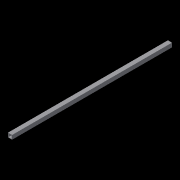
# Autodesk Inventor part: Bumper Rail Side
Saved by Autodesk Inventor 2014 SP1 (Build 180222100, 222)
## iProperties
Created: 2013-11-29
Part Number: Bumper Rail Side
Material: Generic
Document SubType Name: Modeling
Designer: Rauhul Varma
Mass: 82.3834 g
Surface Area: 1040.12 cm^2
Volume: 82.3834 cm^3
Density: 1 g/cm^3
Appearance: Default
Author: Rauhul Varma
Autodesk Inventor part; units mm, degrees
ref_plane "YZ Plane" through (0, 0, 0) normal (1, 0, 0) x (0, 1, 0)
ref_plane "XZ Plane" through (0, 0, 0) normal (0, 1, 0) x (-1, 0, 0)
ref_plane "XY Plane" through (0, 0, 0) normal (0, 0, 1) x (1, 0, 0)
sketch "Sketch1" plane through (0, 0, 0) normal (0, 0, 1) x (1, 0, 0)
  line L0 (0, 0) -> (19.05, 0)
  line L1 (19.05, 0) -> (19.05, 19.05)
  line L2 (19.05, 19.05) -> (0, 19.05)
  line L3 (0, 19.05) -> (0, 0)
  line L4 (17.4625, 17.4625) -> (1.5875, 17.4625)
  line L5 (1.5875, 17.4625) -> (1.5875, 1.5875)
  line L6 (1.5875, 1.5875) -> (17.4625, 1.5875)
  line L7 (17.4625, 1.5875) -> (17.4625, 17.4625)
  dimension "d0" = 19.05
  dimension "d1" = 19.05
  dimension "d2" = 1.5875
  dimension "d3" = 1.5875
  dimension "d4" = 1.5875
  dimension "d5" = 1.5875
  constraints: 16 end point, 4 parallel, 2 horizontal, 2 perpendicular
  measures "d0" distance of L2.end L0.start
  measures "d1" distance of L0.start L0.end
  measures "d2" distance between parallel lines of L2 L4
  measures "d3" distance between parallel lines of L1 L7
  measures "d4" distance between parallel lines of L3 L5
  measures "d5" distance between parallel lines of L0 L6
extrude "Extrusion1" add sketch "Sketch1" along normal blind 742.95
equation "\"d3\" = d2"
equation "\"d4\" = d2"
equation "\"d5\" = d3"
body "Solid1"
